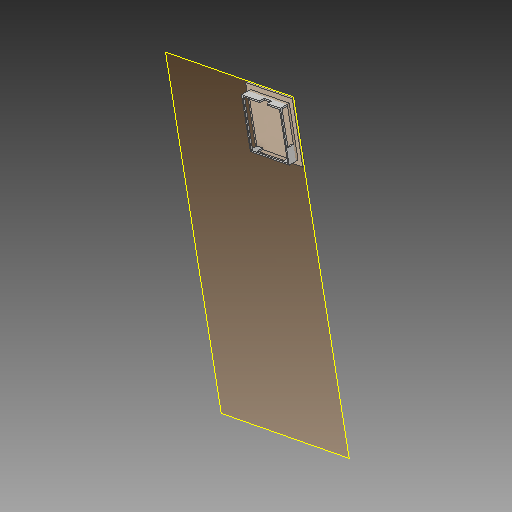
# Autodesk Inventor part: Syno
Saved by Autodesk Inventor 2019 (Build 230136000, 136)
## iProperties
Created: 2020-03-13
Part Number: Syno
Material: Generic
Document SubType Name: Modeling
Designer: Pulag
Mass: 30.5964 g
Surface Area: 158.159 cm^2
Volume: 30.5964 cm^3
Density: 1 g/cm^3
Appearance: Default
Author: Pulag
Autodesk Inventor part; units mm, degrees
ref_plane "YZ Plane" through (0, 0, 0) normal (1, 0, 0) x (0, 1, 0)
ref_plane "XZ Plane" through (0, 0, 0) normal (0, 1, 0) x (-1, 0, 0)
ref_plane "XY Plane" through (0, 0, 0) normal (0, 0, 1) x (1, 0, 0)
ref_plane "Work Plane1" through (80.3117, 823.0211, 0) normal (0, 0, 1) x (0.9814259, 0.1918418, 0)
sketch "Sketch1" plane through (80.3117, 823.0211, 0) normal (0, 0, 1) x (0.9814259, 0.1918418, 0)
  line L0 (98.9183, 339.573) -> (44.3184, 339.573)
  line L1 (44.3184, 339.573) -> (44.3184, 276.403)
  line L2 (44.3184, 276.403) -> (98.9183, 276.403)
  line L3 (98.9183, 276.403) -> (98.9183, 339.573)
  line L4 (98.9183, 339.573) -> (44.3184, 276.403)
  line L5 (42.6184, 341.488) -> (100.6184, 341.488)
  line L6 (100.6184, 341.488) -> (100.6184, 274.488)
  line L7 (100.6184, 274.488) -> (42.6184, 274.488)
  line L8 (42.6184, 274.488) -> (42.6184, 341.488)
  line L9 (42.6184, 341.488) -> (100.6184, 274.488) construction
  line L10 (100.6184, 341.488) -> (42.6184, 274.488) construction
  line L11 (98.9183, 339.573) -> (44.3184, 339.573)
  line L12 (44.3184, 339.573) -> (44.3184, 276.403)
  line L13 (44.3184, 276.403) -> (98.9183, 276.403)
  line L14 (98.9183, 276.403) -> (98.9183, 339.573)
  line L15 (98.9183, 339.573) -> (44.3184, 276.403)
  line L16 (42.6184, 341.488) -> (100.6184, 341.488)
  line L17 (100.6184, 341.488) -> (100.6184, 274.488)
  line L18 (100.6184, 274.488) -> (42.6184, 274.488)
  line L19 (42.6184, 274.488) -> (42.6184, 341.488)
  line L20 (42.6184, 341.488) -> (100.6184, 274.488) construction
  line L21 (100.6184, 341.488) -> (42.6184, 274.488) construction
  point P0 (-236.7099, -792.3271)
  point P1 (71.6184, 307.988)
  point P2 (0, 0)
  point P3 (71.6184, 307.988)
  dimension "d0" = 58
  dimension "d1" = 67
  dimension "d2" = 58
  dimension "d3" = 67
  constraints: 44 end point, 8 parallel, 6 midpoint, 4 horizontal, 4 perpendicular, 4 other
  measures "d0" distance of L6.end L7.end
  measures "d1" distance of L5.end L6.end
  measures "d2" distance of L17.end L18.end
  measures "d3" distance of L16.end L17.end
sketch "Sketch2" plane through (80.3117, 823.0211, 0) normal (0, 0, 1) x (0.9814259, 0.1918418, 0)
  line L0 (98.9183, 339.573) -> (44.3184, 339.573)
  line L1 (44.3184, 339.573) -> (44.3184, 276.403)
  line L2 (44.3184, 276.403) -> (98.9183, 276.403)
  line L3 (98.9183, 276.403) -> (98.9183, 339.573)
  line L4 (42.6184, 341.488) -> (100.6184, 341.488)
  line L5 (100.6184, 341.488) -> (100.6184, 274.488)
  line L6 (100.6184, 274.488) -> (42.6184, 274.488)
  line L7 (42.6184, 274.488) -> (42.6184, 341.488)
  line L8 (42.6184, 341.488) -> (100.6184, 274.488) construction
  line L9 (100.6184, 341.488) -> (42.6184, 274.488) construction
  line L10 (98.9183, 339.573) -> (44.3184, 339.573)
  line L11 (44.3184, 339.573) -> (44.3184, 276.403)
  line L12 (44.3184, 276.403) -> (98.9183, 276.403)
  line L13 (98.9183, 276.403) -> (98.9183, 339.573)
  line L14 (42.6184, 341.488) -> (100.6184, 341.488)
  line L15 (100.6184, 341.488) -> (100.6184, 274.488)
  line L16 (100.6184, 274.488) -> (42.6184, 274.488)
  line L17 (42.6184, 274.488) -> (42.6184, 341.488)
  line L18 (42.6184, 341.488) -> (100.6184, 274.488) construction
  line L19 (100.6184, 341.488) -> (42.6184, 274.488) construction
  point P0 (-236.7099, -792.3271)
  point P1 (0, 0)
  point P2 (71.6184, 307.988)
  point P3 (0, 0)
  point P4 (71.6184, 307.988)
  dimension "d4" = 58
  dimension "d5" = 67
  dimension "d6" = 58
  dimension "d7" = 67
  constraints: 40 end point, 8 parallel, 4 horizontal, 4 midpoint, 4 perpendicular, 4 other
  measures "d4" distance of L5.end L6.end
  measures "d5" distance of L4.end L5.end
  measures "d6" distance of L15.end L16.end
  measures "d7" distance of L14.end L15.end
extrude "Extrusion1" add sketch "Sketch1" along normal blind 10
extrude "Extrusion3" add sketch "Sketch2" against normal blind 3 contours L3 L2 L1 L0 | L4 L5 L6 L7
sketch "Sketch4" plane through (69.4802, 1100.5867, -3) normal (-0.9814259, -0.1918418, 0) x (0, 0, 1)
  line L0 (3, 65.085) -> (13, 65.085) projected
  line L1 (3, 1.915) -> (13, 1.915) projected
  line L2 (3, 65.085) -> (11, 65.085)
  line L3 (11, 65.085) -> (11, 1.915)
  line L4 (11, 1.915) -> (3, 1.915)
  line L5 (3, 1.915) -> (3, 65.085)
  point P0 (3, -1066.8151)
  dimension "d14" = 8
  constraints: 8 end point, 2 parallel, 1 horizontal, 1 perpendicular, 1 point on line
  measures "d14" distance of L3.end L4.end
extrude "Extrusion4" cut sketch "Sketch4" against normal blind 3
sketch "Sketch5" plane through (126.4029, 1111.7135, -3) normal (0.1918418, -0.9814259, 0) x (0.9814259, 0.1918418, 0)
  line L0 (-56.3, 5) -> (-56.3, 3) projected
  line L1 (-41.56, 9.2) -> (-44.06, 9.2) projected
  line L2 (-14.575, 10) -> (-14.575, 9.2) projected
  line L3 (-9.7, 11) -> (-9.7, 3)
  line L4 (-46.3, 11) -> (-9.7, 11)
  line L5 (-9.7, 3) -> (-46.3, 3)
  line L6 (-58, 3) -> (-1.7, 3) projected
  line L7 (-46.3, 11) -> (-43.3, 11)
  line L8 (-43.3, 3) -> (-46.3, 3)
  line L9 (-46.3, 11) -> (-49.3, 11)
  line L10 (-49.3, 11) -> (-49.3, 3)
  line L11 (-49.3, 3) -> (-46.3, 3)
  point P0 (-337.3282, 3)
  dimension "d22" = 8
  dimension "d24" = 8
  dimension "d33" = 3
  dimension "d34" = 3
  constraints: 16 end point, 3 horizontal, 3 parallel, 2 point on line, 1 perpendicular, 1 other
  measures "d22" distance of L4.start L5.end
  measures "d24" distance of L3.end L3.start
  measures "d33" distance of L8.start L8.end
  measures "d34" distance of L11.end L10.end
extrude "Extrusion5" cut sketch "Sketch5" against normal blind 3
sketch "Sketch6" plane through (113.5495, 1177.4691, 10) normal (0.9814259, 0.1918418, 0) x (0, 0, -1)
  line L0 (8, -44.46) -> (3, -44.46)
  line L1 (2, -65.085) -> (2, -1.915) projected
  line L2 (2, -65.085) -> (10, -65.085)
  line L3 (10, -65.085) -> (10, -47.085)
  line L4 (10, -47.085) -> (2, -47.085)
  line L5 (2, -47.085) -> (2, -65.085)
  line L6 (10, -65.085) -> (10, -1.915) projected
  line L7 (2, -47.085) -> (10, -47.085)
  line L8 (10, -47.085) -> (10, -1.915)
  line L9 (10, -1.915) -> (2, -1.915)
  line L10 (2, -1.915) -> (2, -47.085)
  point P0 (10, -1133.8151)
  dimension "d25" = 8
  dimension "d26" = 18
  constraints: 18 end point, 4 parallel, 3 horizontal, 2 perpendicular, 2 other
  measures "d25" distance of L4.end L3.end
  measures "d26" distance of L3.end L2.end
extrude "Extrusion6" cut sketch "Sketch6" against normal blind 3 contours L1 L9 L6 L4
sketch "Sketch7" plane through (56.9942, 1164.4628, 0) normal (0.1918418, -0.9814259, 0) x (0.9814259, 0.1918418, 0)
  line L0 (28.4907, 10.1469) -> (28.4907, 10.1469) projected
  line L1 (27, 8) -> (27, 3.4394)
  line L2 (27, 3.4394) -> (38, 3.4394)
  line L3 (38, 3.4394) -> (38, 8)
  line L4 (38, 3.4394) -> (27, 3.4394)
  line L5 (27, 3.4394) -> (27, 13.4394)
  line L6 (27, 13.4394) -> (38, 13.4394)
  line L7 (38, 13.4394) -> (38, 3.4394)
  point P0 (-279.3282, 0)
  point P1 (35.9907, 10.1469)
  dimension "d29" = 11
  dimension "d32" = 10
  constraints: 14 end point, 3 parallel, 1 horizontal, 1 perpendicular, 2 other
  measures "d29" distance of L2.end L1.end
  measures "d32" distance of L4.end L5.end
extrude "Extrusion7" cut sketch "Sketch7" against normal blind 3
sketch "Sketch8" plane through (80.3117, 823.0211, -3) normal (0, 0, -1) x (-0.9814259, -0.1918418, 0)
  line L0 (-42.6184, 341.488) -> (-100.6184, 341.488) projected
  line L1 (-100.6184, 341.488) -> (-100.6184, 274.488) projected
  line L2 (-42.6184, 274.488) -> (-42.6184, 341.488) projected
  line L3 (-100.6184, 274.488) -> (-42.6184, 274.488) projected
  line L4 (-106.4184, 348.188) -> (-36.8184, 348.188)
  line L5 (-36.8184, 348.188) -> (-36.8184, 267.788)
  line L6 (-36.8184, 267.788) -> (-106.4184, 267.788)
  line L7 (-106.4184, 267.788) -> (-106.4184, 348.188)
  point P0 (236.7099, -792.3271)
  point P1 (-71.6184, 341.488)
  point P2 (-71.6184, 307.988)
  constraints: 8 end point, 2 parallel, 1 horizontal, 1 midpoint, 1 perpendicular
extrude "Extrusion8" add sketch "Sketch8" along normal blind 3 contours L2 L3 L1 L0 | L4 L5 L6 L7
body "Solid1"
